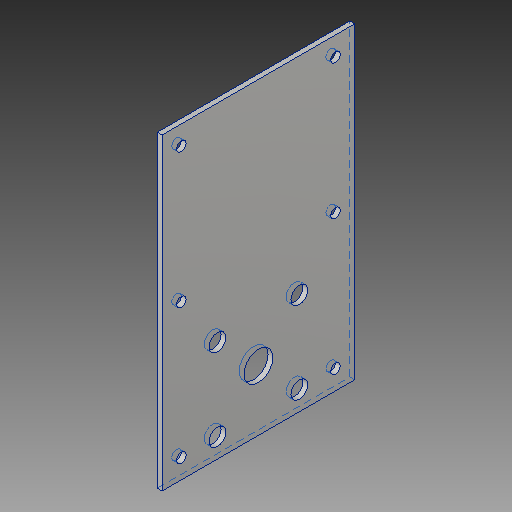
# Autodesk Inventor part: Lateral Plate
Saved by Autodesk Inventor 2019 (Build 230136000, 136)
## iProperties
Created: 2018-09-27
Part Number: Lateral Plate
Material: Aluminum 6061
Document SubType Name: Modeling
Designer: Adhik
Density: 2.7 g/cm^3
Appearance: Aluminum - Flat
Mass: 213.827 g
Surface Area: 529.97 cm^2
Volume: 79.1953 cm^3
Author: Adhik
Autodesk Inventor part; units mm, degrees
ref_plane "YZ Plane" through (0, 0, 0) normal (1, 0, 0) x (0, 1, 0)
ref_plane "XZ Plane" through (0, 0, 0) normal (0, 1, 0) x (-1, 0, 0)
ref_plane "XY Plane" through (0, 0, 0) normal (0, 0, 1) x (1, 0, 0)
sketch "Sketch1" plane through (0, 0, 0) normal (1, 0, 0) x (0, 1, 0)
  line L0 (0, -88.9) -> (0, 88.9) construction
  line L1 (-142.24, 0) -> (142.24, 0) construction
  line L2 (101.6, 63.5) -> (-101.6, 63.5)
  line L3 (-101.6, 63.5) -> (-101.6, -63.5)
  line L4 (-101.6, -63.5) -> (101.6, -63.5)
  line L5 (101.6, -63.5) -> (101.6, 63.5)
  point P0 (0, 0)
  point P1 (0, 63.5)
  point P2 (101.6, 0)
  dimension "d0" = 203.2
  dimension "d1" = 127
  constraints: 8 end point, 2 midpoint, 2 parallel, 2 point on line, 1 horizontal, 1 perpendicular
  measures "d0" distance of L2.start L2.end
  measures "d1" distance of L4.end L2.start
extrude "Extrusion1" add sketch "Sketch1" along normal blind 3.175
sketch "Sketch2" plane through (3.175, 0, 0) normal (1, 0, 0) x (0, 0, -1)
  line L0 (88.9, 0) -> (-88.9, 0) construction
  line L1 (0, -142.24) -> (0, 142.24) construction
  line L2 (-38.1, -23.8125) -> (38.1, -23.8125) construction
  line L3 (38.1, -23.8125) -> (38.1, -100.0125) construction
  line L4 (38.1, -100.0125) -> (-38.1, -100.0125) construction
  line L5 (-38.1, -100.0125) -> (-38.1, -23.8125) construction
  line L6 (-26.9875, -34.925) -> (26.9875, -34.925) construction
  line L7 (26.9875, -34.925) -> (26.9875, -88.9) construction
  line L8 (26.9875, -88.9) -> (-26.9875, -88.9) construction
  line L9 (-26.9875, -88.9) -> (-26.9875, -34.925) construction
  line L10 (-38.1, -61.9125) -> (38.1, -61.9125) construction
  circle A0 centre (-26.9875, -34.925) radius 5.5563
  circle A1 centre (26.9875, -34.925) radius 5.5563
  circle A2 centre (-26.9875, -88.9) radius 5.5563
  circle A3 centre (26.9875, -88.9) radius 5.5563
  line L11 (-63.5, -101.6) -> (63.5, -101.6) construction
  circle A4 centre (0, -61.9125) radius 9.525
  point P0 (0, 0)
  point P1 (0, -23.8125)
  point P2 (0, -34.925)
  point P3 (-26.9875, -61.9125)
  dimension "d4" = 76.2
  dimension "d5" = 53.975
  dimension "d6" = 11.1125
  dimension "d8" = 19.05
  dimension "d29" = 12.7
  constraints: 18 end point, 6 midpoint, 5 centre point, 4 coincident, 4 parallel, 4 perpendicular, 3 equal radius, 3 point on line, 2 horizontal
  measures "d4" distance of L2.end L3.end
  measures "d5" distance of L6.end L7.end
  measures "d6" diameter of A3
  measures "d8" diameter of A4
  measures "d29" distance between parallel lines of L11 L8
extrude "Extrusion2" cut sketch "Sketch2" against normal through all
sketch "Sketch4" plane through (3.175, 0, 0) normal (1, 0, 0) x (0, 0, -1)
  line L0 (88.9, 0) -> (-88.9, 0) construction
  line L1 (0, -144.4625) -> (0, 144.4625) construction
  line L2 (-63.5, 101.6) -> (-38.1, 101.6) construction
  line L3 (-38.1, 101.6) -> (-38.1, -101.6) construction
  line L4 (-38.1, -101.6) -> (-63.5, -101.6) construction
  line L5 (-63.5, -101.6) -> (-63.5, 101.6) construction
  line L6 (-50.8, 101.6) -> (-50.8, -101.6) construction
  line L7 (-38.1, 76.2) -> (-63.5, 76.2) construction
  line L8 (-38.1, 88.9) -> (-63.5, 88.9) construction
  circle A0 centre (-50.8, 88.9) radius 3.175
  circle A1 centre (-50.8, 0) radius 3.175
  circle A2 centre (-50.8, -88.9) radius 3.175
  circle A3 centre (50.8, 88.9) radius 3.175
  circle A4 centre (50.8, 0) radius 3.175
  circle A5 centre (50.8, -88.9) radius 3.175
  point P0 (0, 0)
  dimension "d30" = 25.4
  dimension "d31" = 25.4
  dimension "d32" = 6.35
  constraints: 14 end point, 6 centre point, 4 midpoint, 4 point on line, 4 symmetric about line, 3 horizontal, 2 coincident, 2 parallel, 1 equal radius, 1 perpendicular, 1 vertical, 5 other
  measures "d30" distance of L3.end L4.end
  measures "d31" distance between parallel lines of L2 L7
  measures "d32" diameter of A0
extrude "Extrusion4" cut sketch "Sketch4" against normal through all
body "Solid1"
